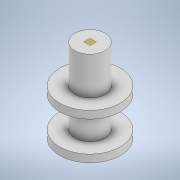
# Autodesk Inventor part: CapstanBottom-ver1-1111-2021
Saved by Autodesk Inventor 2021 (Build 250183000, 183)
## iProperties
Created: 2021-01-28
Part Number: CapstanBottom-ver1-1111-2021
Material: Generic
Document SubType Name: Modeling
Designer: con_c_000
Density: 1 g/cm^3
Appearance: Default
Author: con_c_000
Autodesk Inventor part; units mm, degrees
ref_plane "YZ Plane" through (0, 0, 0) normal (1, 0, 0) x (0, 1, 0)
ref_plane "XZ Plane" through (0, 0, 0) normal (0, 1, 0) x (-1, 0, 0)
ref_plane "XY Plane" through (0, 0, 0) normal (0, 0, 1) x (1, 0, 0)
ref_plane "Work Plane4" through (0, 152.4, 0) normal (0, 1, 0) x (1, 0, 0)
ref_plane "Work Plane5" through (0, 152.4, 0) normal (0, 1, 0) x (1, 0, 0)
ref_plane "Work Plane3" through (0, 152.4, 0) normal (0, -1, 0) x (1, 0, 0)
sketch "Sketch6" plane through (0, 152.4, 0) normal (0, -1, 0) x (1, 0, 0)
  circle A0 centre (0, 0) radius 104.5589 projected
  circle A1 centre (0, 0) radius 50.8
  dimension "d15" = 101.6
  constraints: 1 centre point, 1 coincident
  measures "d15" diameter of A1
extrude "Extrusion6" add sketch "Sketch6" along normal blind 254 contours A1
sketch "Sketch7" plane through (0, -101.6, 0) normal (0, -1, 0) x (1, 0, 0)
  circle A0 centre (0, 0) radius 104.5589 projected
  circle A1 centre (0, 0) radius 101.6
  dimension "d18" = 203.2
  constraints: 1 centre point, 1 coincident
  measures "d18" diameter of A1
extrude "Extrusion7" add sketch "Sketch7" along normal blind 25.4 contours A1
ref_plane "Work Plane1" through (0, 0, 0) normal (0, 1, 0) x (1, 0, 0)
sketch "Sketch8" plane through (0, 0, 0) normal (0, 1, 0) x (1, 0, 0)
  circle A0 centre (0, 0) radius 101.6
  dimension "d22" = 203.2
  constraints: 1 centre point, 1 coincident
  measures "d22" diameter of A0
extrude "Extrusion8" add sketch "Sketch8" along normal blind 25.4
ref_plane "Work Plane2" through (75.376, -18.8821, -44.9646) normal (1, 0, 0) x (0, 1, 0)
sketch "Sketch9" plane through (75.376, -18.8821, -44.9646) normal (1, 0, 0) x (0, 1, 0)
  circle A0 centre (-604.603, 44.9646) radius 12.7
  point P0 (18.8821, 44.9646)
  dimension "d25" = 25.4
  constraints: 1 centre point
  measures "d25" diameter of A0
extrude "Extrusion9" cut sketch "Sketch9" against normal through all
body "Solid1"
